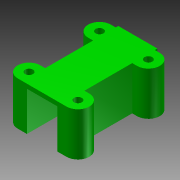
# Autodesk Inventor part: BatteryLatch-Outer
Saved by Autodesk Inventor 2012 (Build 160160000, 160)
## iProperties
Created: 2013-10-13
Part Number: BatteryLatch-Outer
Material: Default
Document SubType Name: Modeling
Designer: joe_000
Density: 1 g/cm^3
screwHoleOffsetFromSide: 0.070 in
screwHoleDiameter: 0.112 in
outerWidth: 0.563 in
outerLength: 1.313 in
wallThickness: 0.063 in
screwOuterDiameter: 0.326 in
screwHoleOffsetFromEnd: 0.000 in
Author: joe_000
Autodesk Inventor part; units mm, degrees
ref_plane "YZ Plane" through (0, 0, 0) normal (1, 0, 0) x (0, 1, 0)
ref_plane "XZ Plane" through (0, 0, 0) normal (0, 1, 0) x (-1, 0, 0)
sketch "Sketch1" plane through (0, 0, 0) normal (0, 0, 1) x (1, 0, 0)
  line L0 (0, 0) -> (1.5875, 0)
  line L1 (1.5875, 0) -> (1.5875, 14.2875)
  line L2 (1.5875, 14.2875) -> (12.7, 14.2875)
  line L3 (12.7, 14.2875) -> (12.7, 0)
  line L4 (12.7, 0) -> (14.2875, 0)
  line L5 (14.2875, 0) -> (14.2875, 15.875)
  line L6 (14.2875, 15.875) -> (0, 15.875)
  line L7 (0, 15.875) -> (0, 0)
  dimension "d1" = 11.1125
  dimension "wallThickness" = 1.5875
  dimension "d4" = 1.5875
  dimension "d5" = 1.5875
  dimension "d6" = 14.2875
  dimension "outerWidth" = 14.2875
  constraints: 16 end point, 5 parallel, 2 collinear, 1 horizontal, 1 perpendicular
  measures "d1" distance of L1.end L2.end
  measures "wallThickness" distance of L3.end L4.end
  measures "d4" distance between parallel lines of L6 L2
  measures "d5" distance of L0.start L0.end
  measures "d6" distance of L2.end L3.end
  measures "outerWidth" distance of L5.end L6.end
extrude "Extrusion1" add sketch "Sketch1" along normal blind 33.3375
sketch "Sketch2" plane through (0, 0, 0) normal (0, 0, -1) x (-1, 0, 0)
  line L0 (0, 15.875) -> (0, 0) projected
  line L1 (-14.2875, 15.875) -> (0, 15.875) projected
  line L2 (-14.2875, 0) -> (-14.2875, 15.875) projected
  line L3 (-14.2875, 0) -> (0, 0)
  line L4 (-12.7, 14.2875) -> (-12.7, 0) projected
  circle A0 centre (-7.1437, 7.1437) radius 1.905
  dimension "d11" = 3.81
  dimension "d12" = 7.1437
  dimension "d13" = 5.5563
  constraints: 2 end point, 1 centre point, 1 perpendicular
  measures "d11" diameter of A0
  measures "d12" distance from line of L3 A0.centre
  measures "d13" distance from line of L4 A0.centre
extrude "Extrusion3" add sketch "Sketch2" along normal blind 1.5875
sketch "Sketch3" plane through (0, 15.875, 33.3375) normal (0, 1, 0) x (1, 0, 0)
  line L0 (0, 34.925) -> (0, 0) projected
  circle A0 centre (-1.778, 4.1406) radius 1.4224
  line L1 (0, 0) -> (-1.778, 0)
  line L2 (0, 8.2812) -> (-1.778, 8.2812)
  arc A1 (-1.778, 8.2812) -> (-1.778, 0) centre (-1.778, 4.1406) ccw
  line L3 (0, 0) -> (14.2875, 0) projected
  point P0 (0, 33.3375)
  dimension "screwOuterDiameter" = 8.2812
  dimension "d24" = 4.1406
  dimension "d25" = 0
  dimension "screwHoleOffsetFromSide" = 1.778
  dimension "screwHoleDiameter" = 2.8448
  constraints: 4 end point, 2 centre point, 2 point on circle, 2 point on line, 2 vertical alignment, 1 collinear, 1 parallel, 1 perpendicular
  measures "screwOuterDiameter" distance between parallel lines of L1 L2
  measures "d24" radius of A1
  measures "d25" distance of A0.centre A1.centre
  measures "screwHoleOffsetFromSide" distance from line of L0 A0.centre
  measures "screwHoleDiameter" diameter of A0
extrude "Extrusion4" add sketch "Sketch3" against normal blind 15.875
pattern_linear "Rectangular Pattern1" count 2 spacing 25.7175 along (0, 0, -1) of "Extrusion4"
ref_plane "Work Plane1" through (7.1438, 0, 33.3375) normal (-1, 0, 0) x (0, 0, -1)
mirror "Mirror1" about plane through (7.1438, 0, 33.3375) normal (-1, 0, 0) of "Extrusion4", "Rectangular Pattern1"
equation "\"d1\" = plungerWidth + plungerTolerance"
equation "\"d4\" = wallThickness"
equation "\"d5\" = wallThickness"
equation "\"d6\" = plungerHeight + plungerTolerance"
equation "\"outerLength\" = plungerLength + springLength"
equation "\"d12\" = 0.5 * d6"
equation "\"d13\" = 0.5 * d1"
equation "\"d14\" = wallThickness"
equation "\"d24\" = 0.5 * screwOuterDiameter"
equation "\"d28\" = wallThickness + plungerHeight + plungerTolerance"
equation "\"plungerWidth\" = 9.525"
equation "\"plungerTolerance\" = 1.5875"
equation "\"plungerHeight\" = 12.7"
equation "\"plungerLength\" = 12.7"
equation "\"springLength\" = 20.6375"
body "Solid1"
